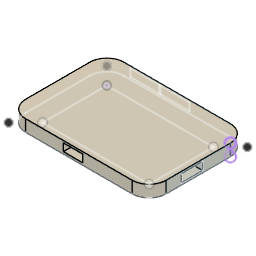
bottom panel (Autodesk Fusion 360 design; units mm, degrees)
part number: 2026-06-26-14-21-11-008
Autodesk Fusion 360 part; units mm, degrees
sketch "Sketch1" plane through (0, 0, 0) normal (0, 1, 0) x (1, 0, 0)
  line L0 (0, 0) -> (63, 0)
  line L1 (63, 0) -> (63, -38)
  line L2 (63, -38) -> (0, -38)
  line L3 (0, -38) -> (0, 0)
  line L4 (0, 10) -> (63, 10)
  line L5 (73, 0) -> (73, -38)
  line L6 (63, -48) -> (0, -48)
  line L7 (-10, -38) -> (-10, 0)
  arc A0 (-10, -38) -> (0, -48) centre (0, -38) ccw
  arc A1 (63, -48) -> (73, -38) centre (63, -38) ccw
  arc A2 (0, 10) -> (-10, 0) centre (0, 0) ccw
  arc A3 (73, 0) -> (63, 10) centre (63, 0) ccw
  point P0 (-10, 10)
  point P1 (73, 10)
  point P2 (-10, -48)
  dimension "d1" = 63
  dimension "d2" = 38
  dimension "d3" = 83
  dimension "d4" = 58
  dimension "d5" = 10
  dimension "d6" = 10
  dimension "d7" = 10
  dimension "d8" = 10
  dimension "d9" = 10
  constraint horizontal L0
  constraint vertical L1
  constraint horizontal L2
  constraint vertical L3
  constraint coincident L0.start L3.end
  constraint horizontal L4
  constraint vertical L5
  constraint horizontal L6
  constraint vertical L7
  constraint coincident P2 L6
  constraint coincident P2 L7
  constraint tangent L6 A0
  constraint tangent L7 A0
  constraint tangent L5 A1
  constraint tangent L6 A1
  constraint equal A0 A1
  constraint coincident P0 L4
  constraint coincident P0 L7
  constraint tangent L4 A2
  constraint tangent L7 A2
  constraint coincident P1 L4
  constraint coincident P1 L5
  constraint tangent L4 A3
  constraint tangent L5 A3
  measures "d1" distance of L0.start L0.end
  measures "d2" distance of L0.start L2.end
  measures "d3" distance of P0 P1
  measures "d4" distance of P0 P2
  measures "d5" distance of L3 L7
  measures "d6" distance of L0 L4
  measures "d7" radius of A0
  measures "d8" radius of A2
  measures "d9" radius of A3
extrude "Extrude1" add sketch "Sketch1" along normal blind 3 contours L0 L1 L2 L3
extrude "Extrude2" add sketch "Sketch1" along normal blind 3
extrude "Extrude3" add 1 faces at (21, 3, 28.6667) along direction (0, 1, 0) blind 4
extrude "Extrude4" cut sketch "Sketch1" along normal blind 6 contours L0 L1 L2 L3
sketch "Sketch3" plane through (0, 0, -10) normal (0, 0, -1) x (-1, 0, 0)
  line L0 (-63, 0) -> (0, 0)
  line L1 (0, 0) -> (0, 7)
  line L2 (0, 7) -> (-63, 7)
  line L3 (-63, 7) -> (-63, 0)
  line L4 (-3.9, 1.3) -> (-20.9, 1.3)
  line L5 (-20.9, 1.3) -> (-20.9, 5.8)
  line L6 (-20.9, 5.8) -> (-3.9, 5.8)
  line L7 (-3.9, 5.8) -> (-3.9, 1.3)
  line L8 (-21.8, 1.3) -> (-38.8, 1.3)
  line L9 (-38.8, 1.3) -> (-38.8, 5.8)
  line L10 (-38.8, 5.8) -> (-21.8, 5.8)
  line L11 (-21.8, 5.8) -> (-21.8, 1.3)
  dimension "d18" = 17
  dimension "d19" = 4.5
  dimension "d20" = 1.2
  dimension "d21" = 3.9
  dimension "d22" = 17
  dimension "d23" = 4.5
  dimension "d24" = 1.2
  dimension "d25" = 0.9
  constraint horizontal L4
  constraint vertical L5
  constraint horizontal L6
  constraint vertical L7
  constraint horizontal L8
  constraint vertical L9
  constraint horizontal L10
  constraint vertical L11
  measures "d18" distance of L4.start L4.end
  measures "d19" distance of L4.start L6.end
  measures "d20" distance of L2 L6
  measures "d21" distance of L1 L7
  measures "d22" distance of L8.start L8.end
  measures "d23" distance of L8.start L10.end
  measures "d24" distance of L2 L10
  measures "d25" distance of L5 L11
extrude "Extrude5" cut sketch "Sketch3" against normal blind 10 contours L4 L5 L6 L7
sketch "Sketch4" plane through (73, 0, 0) normal (1, 0, 0) x (0, 0, -1)
  line L0 (-38, 0) -> (0, 0)
  line L1 (0, 0) -> (0, 7)
  line L2 (0, 7) -> (-38, 7)
  line L3 (-38, 7) -> (-38, 0)
  line L4 (-16.5, 1.3) -> (-29, 1.3)
  line L5 (-29, 1.3) -> (-29, 5.8)
  line L6 (-29, 5.8) -> (-16.5, 5.8)
  line L7 (-16.5, 5.8) -> (-16.5, 1.3)
  line L8 (0, 0) -> (0, 7)
  dimension "d28" = 12.5
  dimension "d29" = 4.5
  dimension "d30" = 1.2
  dimension "d31" = 16.5
  constraint horizontal L4
  constraint vertical L5
  constraint horizontal L6
  constraint vertical L7
  measures "d28" distance of L4.start L4.end
  measures "d29" distance of L4.start L6.end
  measures "d30" distance of L2 L6
  measures "d31" distance of L7 L8
extrude "Extrude6" cut sketch "Sketch4" against normal blind 10 contours L4 L5 L6 L7
sketch "Sketch5" plane through (0, 0, 48) normal (0, 0, 1) x (1, 0, 0)
  line L0 (0, 0) -> (63, 0)
  line L1 (63, 0) -> (63, 7)
  line L2 (63, 7) -> (0, 7)
  line L3 (0, 7) -> (0, 0)
  line L4 (33.7, 1.3) -> (22.3, 1.3)
  line L5 (22.3, 1.3) -> (22.3, 5.8)
  line L6 (22.3, 5.8) -> (33.7, 5.8)
  line L7 (33.7, 5.8) -> (33.7, 1.3)
  dimension "d34" = 11.4
  dimension "d35" = 4.5
  dimension "d36" = 1.2
  dimension "d37" = 29.3
  constraint horizontal L4
  constraint vertical L5
  constraint horizontal L6
  constraint vertical L7
  measures "d34" distance of L4.start L4.end
  measures "d35" distance of L4.start L6.end
  measures "d36" distance of L2 L6
  measures "d37" distance of L1 L7
extrude "Extrude7" cut sketch "Sketch3" against normal blind 10 contours L8 L9 L10 L11
extrude "Extrude8" cut sketch "Sketch5" against normal blind 10 contours L4 L5 L6 L7
